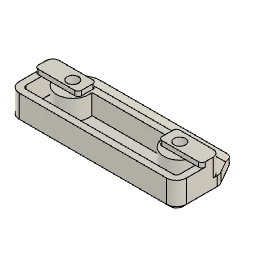
Rear Bottom Mid Clip (Autodesk Fusion 360 design; units mm, degrees)
Autodesk Fusion 360 part; units mm, degrees
note: some values were not read from the file. Chosen so that the rebuilt part matches the saved one: which face or edge a step refers to; which pieces of a blend or face edit are solid. Set by a fixed rule: which sketch regions a step uses.
sketch "Sketch1" plane through (0, 0, 0) normal (0, 0, 1) x (1, 0, 0)
  line L0 (25, 6.5) -> (-25, 6.5)
  line L1 (-25, 6.5) -> (-25, -6.5)
  line L2 (-25, -6.5) -> (25, -6.5)
  line L3 (25, -6.5) -> (25, 6.5)
  line L4 (25, 6.5) -> (-25, -6.5) construction
  line L5 (-25, 6.5) -> (25, -6.5) construction
  line L6 (-16, 3.5) -> (16, 3.5) construction
  line L7 (0, 0) -> (0, 3.5) construction
  circle A0 centre (-16, 3.5) radius 1.7
  circle A1 centre (16, 3.5) radius 1.7
  dimension "d1" = 50
  dimension "d2" = 13
  dimension "d4" = 10
  dimension "d5" = 9
  dimension "d6" = 3.4
  constraint horizontal L0
  constraint perpendicular L0 L1
  constraint parallel L0 L2
  constraint parallel L1 L3
  constraint coincident L4 L7.start
  constraint coincident L5 L7.start
  constraint coincident L7.start origin
  constraint horizontal L6
  constraint vertical L7
  constraint midpoint L6 L7.end
  constraint coincident L6.start A0.centre
  constraint coincident L6.end A1.centre
  constraint equal A0 A1
  measures "d1" distance of L1.end L2.end
  measures "d2" distance of L0.end L1.end
  measures "d4" distance of L2 L7.end
  measures "d5" distance of L1 L6.start
  measures "d6" diameter of A0
extrude "Extrude1" add sketch "Sketch1" along normal blind 4
sketch "Sketch2" plane through (0, 0, 0) normal (0, 0, -1) x (1, 0, 0)
  circle A0 centre (-16, -3.5) radius 1.7
  circle A1 centre (16, -3.5) radius 1.7
  line L0 (25, -6.5) -> (25, 6.5)
  line L1 (25, 6.5) -> (-25, 6.5)
  line L2 (-25, 6.5) -> (-25, -6.5)
  line L3 (-25, -6.5) -> (25, -6.5)
  line L4 (25, -6.5) -> (20.3812, -14.5)
  line L5 (20.3812, -14.5) -> (-20.3812, -14.5)
  line L6 (-20.3812, -14.5) -> (-25, -6.5)
  line L7 (0, 0) -> (0, -14.5) construction
  dimension "d9" = 60
  dimension "d10" = 8
  constraint coincident L0.start L3.end
  constraint perpendicular L0 L5
  constraint coincident L2.end L3.start
  constraint coincident L7.start origin
  constraint perpendicular L3 L7
  constraint midpoint L5 L7.end
  measures "d9" angle of L3 L4
  measures "d10" distance of L3 L5
extrude "Extrude2" add sketch "Sketch2" along normal blind 4
sketch "Sketch3" plane through (25, 0, 0) normal (1, 0, 0) x (0, 1, 0)
  line L0 (6.5, 0) -> (6.5, 4)
  line L1 (6.5, 4) -> (-6.5, 4)
  line L2 (-6.5, 4) -> (-6.5, -4)
  line L3 (-6.5, -4) -> (6.5, -4)
  line L4 (6.5, -4) -> (6.5, 0)
  line L5 (14.5, 0) -> (6.5, 0)
  line L6 (6.5, 0) -> (6.5, -4)
  line L7 (6.5, -4) -> (14.5, -4)
  line L8 (14.5, -4) -> (14.5, 0)
  line L9 (10.5, 0) -> (14.5, -1.6)
  dimension "d13" = 1.6
  dimension "d14" = 4
  constraint coincident L5 L9.start
  constraint coincident L8 L9.end
  measures "d13" distance of L5.start L9.end
  measures "d14" distance of L5.start L9.start
extrude "Extrude3" cut sketch "Sketch3" against normal through all contours L5 L8 L9
fillet "Fillet2" radius 2 2 edges at (-25, 6.5, 2) (25, 6.5, 2)
fillet "Fillet1" radius 3 6 edges at (25, -6.5, 0) (-25, -6.5, 0) (-20.3812, 14.5, -2.8) (20.3812, 14.5, -2.8) (-25, 6.5, -2) (25, 6.5, -2)
sketch "Sketch4" plane through (0, 0, -4) normal (0, 0, -1) x (1, 0, 0)
  arc A0 (24.5981, -7.1962) -> (25, -5.6962) centre (22, -5.6962) ccw
  line L0 (25, -5.6962) -> (25, 3.5)
  arc A1 (25, 3.5) -> (22, 6.5) centre (22, 3.5) ccw
  line L1 (22, 6.5) -> (-22, 6.5)
  arc A2 (-22, 6.5) -> (-25, 3.5) centre (-22, 3.5) ccw
  line L2 (-25, 3.5) -> (-25, -5.6962)
  arc A3 (-25, -5.6962) -> (-24.5981, -7.1962) centre (-22, -5.6962) ccw
  line L3 (-24.5981, -7.1962) -> (-21.2472, -13)
  arc A4 (-21.2472, -13) -> (-18.6491, -14.5) centre (-18.6491, -11.5) ccw
  line L4 (-18.6491, -14.5) -> (18.6491, -14.5)
  arc A5 (18.6491, -14.5) -> (21.2472, -13) centre (18.6491, -11.5) ccw
  line L5 (21.2472, -13) -> (24.5981, -7.1962)
  circle A6 centre (-16, -3.5) radius 1.7
  circle A7 centre (16, -3.5) radius 1.7
  circle A8 centre (16, -3.5) radius 3
  circle A9 centre (-16, -3.5) radius 3
  dimension "d20" = 6
  constraint concentric A7 A8
  constraint concentric A6 A9
  constraint equal A8 A9
  measures "d20" diameter of A8
extrude "Extrude4" cut sketch "Sketch4" against normal up to surface (4.2 mm away) contours A8 | A9
sketch "Sketch8" plane through (0, 0, 0.2) normal (0, 0, -1) x (1, 0, 0)
  circle A0 centre (16, -3.5) radius 1.7
  circle A1 centre (16, -3.5) radius 3
  circle A2 centre (-16, -3.5) radius 1.7
  circle A3 centre (-16, -3.5) radius 3
  line L0 (18.4718, -5.2) -> (13.5282, -5.2)
  line L1 (18.4718, -1.8) -> (13.5282, -1.8)
  line L2 (-13.5282, -5.2) -> (-18.4718, -5.2)
  line L3 (-13.5282, -1.8) -> (-13.704, -1.8)
  line L4 (-13.704, -1.8) -> (-18.4718, -1.8)
  constraint coincident A1 L0.start
  constraint coincident A1 L0.end
  constraint horizontal L0
  constraint coincident A1 L1.start
  constraint coincident A1 L1.end
  constraint parallel L0 L1
  constraint coincident A3 L2.start
  constraint coincident A3 L2.end
  constraint parallel L1 L2
  constraint coincident A3 L3.start
  constraint parallel L2 L3
  constraint coincident A3 L4.end
  constraint parallel L2 L4
  constraint tangent A0 L0
  constraint tangent A0 L1
  constraint tangent A2 L4
  constraint tangent A2 L2
extrude "Extrude9" add sketch "Sketch8" along normal blind 0.2 contours A1 L1 | A1 L0 | A3 L3 L4 | A3 L2
sketch "Sketch10" plane through (0, 0, 0.2) normal (0, 0, -1) x (1, 0, 0)
  line L0 (18.4718, -1.8) -> (16, -1.8)
  arc A0 (16, -5.2) -> (16, -1.8) centre (16, -3.5) ccw
  line L1 (16, -5.2) -> (18.4718, -5.2)
  arc A1 (18.4718, -5.2) -> (18.4718, -1.8) centre (16, -3.5) ccw
  line L2 (16, -1.8) -> (13.5282, -1.8)
  arc A2 (13.5282, -1.8) -> (13.5282, -5.2) centre (16, -3.5) ccw
  line L3 (13.5282, -5.2) -> (16, -5.2)
  arc A3 (16, -1.8) -> (16, -5.2) centre (16, -3.5) ccw
  line L4 (-16, -5.2) -> (-13.5282, -5.2)
  arc A4 (-13.5282, -5.2) -> (-13.5282, -1.8) centre (-16, -3.5) ccw
  line L5 (-13.5282, -1.8) -> (-16, -1.8)
  arc A5 (-16, -5.2) -> (-16, -1.8) centre (-16, -3.5) ccw
  line L6 (-18.4718, -5.2) -> (-16, -5.2)
  arc A6 (-16, -1.8) -> (-16, -5.2) centre (-16, -3.5) ccw
  line L7 (-16, -1.8) -> (-18.4718, -1.8)
  arc A7 (-18.4718, -1.8) -> (-18.4718, -5.2) centre (-16, -3.5) ccw
  line L8 (17.7, -5.2) -> (17.7, -1.8)
  line L9 (14.3, -5.2) -> (14.3, -1.8)
  line L10 (-14.3, -5.2) -> (-14.3, -1.8)
  line L11 (-17.7, -5.2) -> (-17.7, -1.8)
  constraint coincident L1 L8.start
  constraint coincident L0 L8.end
  constraint perpendicular L0 L8
  constraint coincident L3 L9.start
  constraint coincident L2 L9.end
  constraint perpendicular L2 L9
  constraint coincident L4 L10.start
  constraint coincident L5 L10.end
  constraint perpendicular L5 L10
  constraint coincident L6 L11.start
  constraint coincident L7 L11.end
  constraint perpendicular L7 L11
  constraint tangent A0 L8
  constraint tangent A3 L9
  constraint tangent A5 L10
  constraint tangent A6 L11
extrude "Extrude10" cut sketch "Sketch10" against normal blind 0.2 contours L0 A0 L8 | L2 A3 L9 | A0 L1 L8 | L3 A3 L9 | L4 A5 L10 | L6 A6 L11 | L5 A5 L10 | A6 L7 L11
chamfer "Chamfer1" distance 1.2 angle 45 12 edges at (-20.1491, 14.0981, -4) (-22.9226, 10.0981, -4) (-24.8978, 6.4726, -4) (-25, 1.0981, -4) (-24.1213, -5.6213, -4) (0, -6.5, -4) (24.1213, -5.6213, -4) (25, 1.0981, -4) (24.8978, 6.4726, -4) (22.9226, 10.0981, -4) (20.1491, 14.0981, -4) (0, 14.5, -4)
shell "Shell1" thickness 2 removed faces 1 at (-4.98, -3.6097, 4)
sketch "Sketch11" plane through (0, 0, 4) normal (0, 0, 1) x (-1, 0, 0)
  line L0 (23, 3.5) -> (23, -4.5)
  line L1 (23, -4.5) -> (19.5623, -4.5)
  arc A0 (19.5623, -4.5) -> (12.4377, -4.5) centre (16, -3.5) ccw
  line L2 (12.4377, -4.5) -> (-12.4377, -4.5)
  arc A1 (-12.4377, -4.5) -> (-19.5623, -4.5) centre (-16, -3.5) ccw
  line L3 (-19.5623, -4.5) -> (-23, -4.5)
  line L4 (-23, -4.5) -> (-23, 3.5)
  arc A2 (-22, 4.5) -> (-23, 3.5) centre (-22, 3.5) ccw
  line L5 (-22, 4.5) -> (22, 4.5)
  arc A3 (23, 3.5) -> (22, 4.5) centre (22, 3.5) ccw
  circle A4 centre (-16, -3.5) radius 1.7
  circle A5 centre (16, -3.5) radius 1.7
  arc A6 (25, 3.5) -> (22, 6.5) centre (22, 3.5) ccw
  line L6 (22, 6.5) -> (-22, 6.5)
  arc A7 (-22, 6.5) -> (-25, 3.5) centre (-22, 3.5) ccw
  line L7 (-25, 3.5) -> (-25, -4.5)
  arc A8 (-25, -4.5) -> (-23, -6.5) centre (-23, -4.5) ccw
  line L8 (-23, -6.5) -> (23, -6.5)
  arc A9 (23, -6.5) -> (25, -4.5) centre (23, -4.5) ccw
  line L9 (25, -4.5) -> (25, 3.5)
  circle A10 centre (16, -3.5) radius 5.3
  circle A11 centre (-16, -3.5) radius 5.3
  dimension "d41" = 10.6
  constraint concentric A0 A10
  constraint concentric A1 A11
  constraint equal A10 A11
  measures "d41" diameter of A10
extrude "Extrude11" add sketch "Sketch11" against normal up to surface (8 mm away) contours L1 A0 L2 A10 | L2 A1 L3 A11
sketch "Sketch7" plane through (0, 0, 4) normal (0, 0, 1) x (-1, 0, 0)
  line L0 (23, -4.5) -> (21.2048, -4.5)
  line L1 (-23, -4.5) -> (-23, 3.5)
  arc A0 (-22, 4.5) -> (-23, 3.5) centre (-22, 3.5) ccw
  line L2 (-22, 4.5) -> (22, 4.5)
  arc A1 (23, 3.5) -> (22, 4.5) centre (22, 3.5) ccw
  line L3 (23, 3.5) -> (23, -4.5)
  circle A2 centre (-16, -3.5) radius 1.7
  circle A3 centre (16, -3.5) radius 1.7
  arc A4 (25, 3.5) -> (22, 6.5) centre (22, 3.5) ccw
  line L4 (22, 6.5) -> (-22, 6.5)
  arc A5 (-22, 6.5) -> (-25, 3.5) centre (-22, 3.5) ccw
  line L5 (-25, 3.5) -> (-25, -4.5)
  arc A6 (-25, -4.5) -> (-23, -6.5) centre (-23, -4.5) ccw
  line L6 (-23, -6.5) -> (23, -6.5)
  arc A7 (23, -6.5) -> (25, -4.5) centre (23, -4.5) ccw
  line L7 (25, -4.5) -> (25, 3.5)
  line L8 (-25, -1.1) -> (-12, -1.1)
  line L9 (-12, -1.1) -> (-12, -6.5)
  line L10 (12, -6.5) -> (12, -1.1)
  line L11 (12, -1.1) -> (25, -1.1)
  arc A8 (21.2048, -4.5) -> (10.7952, -4.5) centre (16, -3.5) ccw
  line L12 (10.7952, -4.5) -> (-10.7952, -4.5)
  arc A9 (-10.7952, -4.5) -> (-21.2048, -4.5) centre (-16, -3.5) ccw
  line L13 (-21.2048, -4.5) -> (-23, -4.5)
  dimension "d31" = 5.4
  dimension "d32" = 13
  constraint perpendicular L5 L8
  constraint coincident L6 L9.end
  constraint perpendicular L6 L9
  constraint coincident L6 L10.start
  constraint perpendicular L6 L10
  constraint coincident L7 L11.end
  constraint perpendicular L7 L11
  constraint equal L8 L11
  constraint coincident L5 L8.start
  constraint equal L9 L10
  measures "d31" distance of L8.end L9.end
  measures "d32" distance of L8.start L8.end
extrude "Extrude8" add sketch "Sketch7" along normal blind 1.4 contours L0 L3 L6 A7 L7 L10 L11 A8 | L0 L3 L11 A8 | L1 L5 A6 L6 L8 L9 A9 L13 | L1 L8 A9 L13
fillet "Fillet4" radius 1 6 edges at (-12, 1.1, 4.7) (-12, 6.5, 4.7) (12, 1.1, 4.7) (12, 6.5, 4.7) (-25, 1.1, 4.7) (25, 1.1, 4.7)
move_face "OffsetFaces1" offset -0.5 2 faces at (-10.7246, 4.0095, 1.3333) (10.7246, 4.0095, 1.3333)
